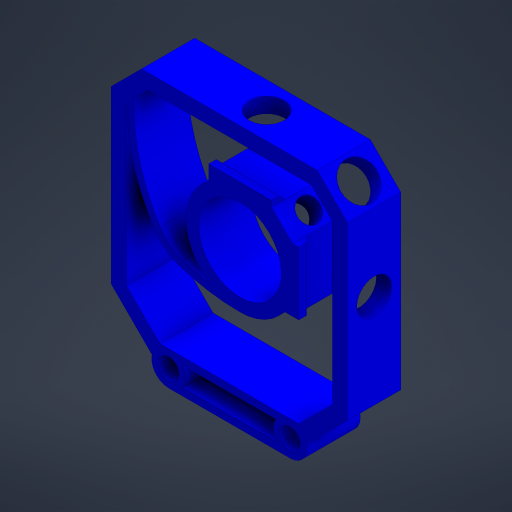
# Autodesk Inventor part: SM05 Lense Holder (V5)
Saved by Autodesk Inventor 2023.4 (Build 274418000, 418)
## iProperties
Created: 2022-07-25
Part Number: SM05 Lense Holder (V5)
Material: Generic
Document SubType Name: Modeling
Designer: xSibe
Density: 1 g/cm^3
Appearance: Plastic Blue
Author: xSibe
Autodesk Inventor part; units mm, degrees
ref_plane "YZ Plane" through (0, 0, 0) normal (1, 0, 0) x (0, 1, 0)
ref_plane "XZ Plane" through (0, 0, 0) normal (0, 1, 0) x (-1, 0, 0)
sketch "Sketch1" plane through (0, 0, 0) normal (0, 0, 1) x (1, 0, 0)
  circle A0 centre (10, 3.85) radius 1.5625
  circle A1 centre (-10, 3.85) radius 1.5625
  line L0 (-16.9, 0) -> (16.9, 0)
  line L1 (16.9, 0) -> (16.9, 7.7)
  line L2 (-16.9, 7.7) -> (16.9, 7.7)
  line L3 (-16.9, 0) -> (-16.9, 7.7)
  circle A2 centre (-10, 3.85) radius 2.8125
  circle A3 centre (10, 3.85) radius 2.8125
  line L4 (-10, 6.6625) -> (10, 6.6625)
  line L5 (10, 1.0375) -> (-10, 1.0375)
  line L6 (-10, 2.2875) -> (10, 2.2875)
  line L7 (-10, 5.4125) -> (10, 5.4125)
  line L8 (-17.05, 7.7) -> (-17.05, 42.1)
  line L9 (17.05, 7.7) -> (17.05, 42.1)
  line L10 (-17.05, 24.9) -> (17.05, 24.9)
  line L11 (0, 24.9) -> (1.767767, 26.667767)
  line L12 (0, 24.9) -> (2.5, 24.9) construction
  circle A4 centre (1.767767, 26.667767) radius 6.78375
  circle A5 centre (1.767767, 26.667767) radius 6.10875
  circle A6 centre (1.767767, 26.667767) radius 8.90875
  line L13 (1.767767, 26.667767) -> (1.767767, 35.576517)
  line L14 (1.767767, 35.576517) -> (1.767767, 35.076517)
  line L15 (-3.419733, 33.826517) -> (6.955267, 33.826517)
  line L16 (6.955267, 33.826517) -> (6.955267, 36.326517)
  line L17 (6.955267, 36.326517) -> (-3.419733, 36.326517)
  line L18 (-3.419733, 36.326517) -> (-3.419733, 33.826517)
  line L19 (-3.419733, 33.826517) -> (6.955267, 36.326517) construction
  line L20 (6.955267, 33.826517) -> (-3.419733, 36.326517) construction
  line L21 (1.767767, 26.667767) -> (8.067204, 32.967204)
  line L22 (8.067204, 32.967204) -> (7.625263, 32.525263)
  line L23 (10.45369, 31.818156) -> (6.918156, 35.35369)
  line L24 (6.918156, 35.35369) -> (4.796836, 33.23237)
  line L25 (4.796836, 33.23237) -> (8.33237, 29.696836)
  line L26 (8.33237, 29.696836) -> (10.45369, 31.818156)
  line L27 (10.45369, 31.818156) -> (4.796836, 33.23237) construction
  line L28 (6.918156, 35.35369) -> (8.33237, 29.696836) construction
  line L29 (10.45369, 31.818156) -> (15.45369, 31.818156) construction
  line L30 (8.926517, 21.480267) -> (8.926517, 31.855267)
  line L31 (8.926517, 31.855267) -> (11.426517, 31.855267)
  line L32 (11.426517, 31.855267) -> (11.426517, 21.480267)
  line L33 (11.426517, 21.480267) -> (8.926517, 21.480267)
  line L34 (1.767767, 35.576517) -> (1.767767, 37.576517)
  line L35 (11.426517, 26.667767) -> (13.426517, 26.667767)
  line L36 (-10.217767, 5.432233) -> (10.217767, 5.432233)
  line L37 (19.467767, 14.682233) -> (19.467767, 39.367767)
  line L38 (14.467767, 44.367767) -> (-14.467767, 44.367767)
  line L39 (-19.467767, 39.367767) -> (-19.467767, 14.682233)
  line L40 (-19.467767, 5.432233) -> (19.467767, 44.367767) construction
  line L41 (19.467767, 5.432233) -> (-19.467767, 44.367767) construction
  line L42 (-10.217767, 5.432233) -> (-19.467767, 14.682233)
  line L43 (10.217767, 5.432233) -> (19.467767, 14.682233)
  line L44 (14.467767, 44.367767) -> (19.467767, 39.367767)
  line L45 (-14.467767, 44.367767) -> (-19.467767, 39.367767)
  line L46 (-15.503301, 46.867767) -> (-21.967767, 40.403301)
  line L47 (-21.967767, 40.403301) -> (-21.967767, 13.646699)
  line L48 (-21.967767, 13.646699) -> (-11.253301, 2.932233)
  line L49 (-11.253301, 2.932233) -> (11.253301, 2.932233)
  line L50 (11.253301, 2.932233) -> (21.967767, 13.646699)
  line L51 (21.967767, 13.646699) -> (21.967767, 40.403301)
  line L52 (21.967767, 40.403301) -> (15.503301, 46.867767)
  line L53 (15.503301, 46.867767) -> (-15.503301, 46.867767)
  line L54 (-13.432233, 41.867767) -> (-16.967767, 38.332233)
  line L55 (-16.967767, 38.332233) -> (-16.967767, 15.717767)
  line L56 (-16.967767, 15.717767) -> (-9.182233, 7.932233)
  line L57 (-9.182233, 7.932233) -> (9.182233, 7.932233)
  line L58 (9.182233, 7.932233) -> (16.967767, 15.717767)
  line L59 (16.967767, 15.717767) -> (16.967767, 38.332233)
  line L60 (16.967767, 38.332233) -> (13.432233, 41.867767)
  line L61 (13.432233, 41.867767) -> (-13.432233, 41.867767)
  line L62 (16.967767, 15.717767) -> (16.967767, 8.646699)
  line L63 (-16.967767, 15.717767) -> (-16.967767, 12.182233)
  line L64 (-19.467767, 14.682233) -> (-19.467767, 11.146699)
  line L65 (19.467767, 14.682233) -> (19.467767, 11.146699)
  circle A7 centre (-10, 3.85) radius 1.705
  circle A8 centre (10, 3.85) radius 1.707
  line L66 (-10, 6.6625) -> (-11.448034, 6.6625)
  line L67 (10, 6.6625) -> (11.448034, 6.6625)
  line L68 (1.767767, 17.759017) -> (-10.732233, 17.759017)
  line L69 (-10.732233, 17.759017) -> (-10.732233, 20.259017)
  arc A9 (-10.732233, 20.259017) -> (1.767767, 17.759017) centre (1.767767, 50.259017) ccw
  arc A10 (-16.967767, 38.332233) -> (-10.732233, 20.259017) centre (12.341914, 38.332233) ccw
  arc A11 (-15.688595, 39.611405) -> (-9.948301, 21.288407) centre (12.341914, 38.332233) ccw
  arc A12 (-9.948301, 21.288407) -> (-3.451418, 19.447938) centre (1.767767, 50.259017) ccw
  line L70 (-10.732233, 20.259017) -> (-12.188467, 22.291105)
  line L71 (-9.948301, 21.288407) -> (-11.376856, 23.340048)
  arc A13 (-12.188467, 22.291105) -> (-8.426288, 19.399152) centre (-6.171148, 26.226005) ccw
  arc A14 (-11.376856, 23.340048) -> (-7.633596, 20.45672) centre (-5.565218, 27.013474) ccw
  point P0 (0, 0)
  point P1 (-7.661464, 2.2875)
  point P2 (-7.661464, 5.4125)
  point P3 (7.661464, 5.4125)
  point P4 (7.661464, 2.2875)
  point P5 (7.341455, 2.932233)
  point P6 (-7.341455, 2.932233)
  point P7 (-11.185824, 6.40029)
  point P8 (11.185824, 6.40029)
  point P9 (-3.419733, 33.910396)
  point P10 (9.010396, 21.480267)
  point P11 (9.010396, 31.855267)
  point P12 (9.581848, 30.946314)
  point P13 (6.046314, 34.481848)
  point P14 (6.955267, 33.910396)
  point P15 (12.751875, 4.430808)
  point P16 (-12.751875, 4.430808)
  point P17 (5.390983, 33.826517)
  point P18 (-2.842005, 34.542767)
  point P19 (9.642767, 22.057995)
  point P20 (8.926517, 30.290983)
  point P21 (10.676517, 26.667767)
  point P22 (10.416579, 31.855267)
  point P23 (9.642767, 31.277539)
  point P24 (6.377539, 34.542767)
  point P25 (1.767767, 35.576517)
  point P26 (6.955267, 35.316579)
  point P27 (8.067204, 32.967204)
  point P28 (-17.05, 12.264466)
  point P29 (16.967767, 24.9)
  point P30 (17.05, 12.264466)
  point P31 (-16.967767, 24.9)
  point P32 (16.967767, 12.182233)
  point P33 (10.499366, 24.9)
  point P34 (-6.963832, 24.9)
  point P35 (-17.05, 41.785534)
  point P36 (17.05, 41.785534)
  point P37 (7.67477, 5.432233)
  point P38 (-7.67477, 5.432233)
  point P39 (12.485534, 7.7)
  point P40 (-12.485534, 7.7)
  point P41 (6.564603, 31.464603)
  dimension "d0" = 1.25
  dimension "d1" = 1.25
  dimension "d2" = 2.5
  dimension "d3" = 45
  dimension "d4" = 13.5675
  dimension "d5" = 0.675
  dimension "d6" = 2.125
  dimension "d7" = 0.5
  dimension "d8" = 10.375
  dimension "d9" = 2.5
  dimension "d10" = 0.625
  dimension "d11" = 5
  dimension "d12" = 135
  dimension "d13" = 3
  dimension "d14" = 2
  dimension "d15" = 2
  dimension "d16" = 38.93553
  dimension "d17" = 38.93553
  dimension "d18" = 9.25
  dimension "d19" = 9.25
  dimension "d20" = 9.25
  dimension "d21" = 9.25
  dimension "d22" = 5
  dimension "d23" = 5
  dimension "d24" = 5
  dimension "d25" = 5
  dimension "d26" = 2.5
  dimension "d46" = 2.5
  dimension "d48" = 0.1425
  dimension "d49" = 0.1445
  dimension "d50" = 12.5
  dimension "d51" = 2.5
  dimension "d52" = 1.25
  dimension "d53" = 2.5
  dimension "d54" = 2.5
  constraints: 132 end point, 28 point on circle, 19 point on line, 14 tangent, 13 centre point, 13 parallel, 10 midpoint, 8 horizontal, 8 perpendicular, 4 symmetric about line, 2 equal length, 2 vertical, 1 coincident, 15 other
  measures "d0" radial gap between concentric circles of A1 A2
  measures "d1" radial gap between concentric circles of A0 A3
  measures "d2" distance of L11.start L11.end
  measures "d3" angle of L12 L11
  measures "d4" diameter of A4
  measures "d5" radial gap between concentric circles of A4 A5
  measures "d6" radial gap between concentric circles of A4 A6
  measures "d7" distance of L13.end L14.end
  measures "d8" distance of L17.end L16.end
  measures "d9" distance of L16.end L15.end
  measures "d10" distance of L21.end L22.end
  measures "d11" distance of L23.start L23.end
  measures "d12" angle of L29 L23
  measures "d13" distance of L24.end L23.end
  measures "d14" distance of L13.end L34.end
  measures "d15" distance of L35.start L35.end
  measures "d16" distance of L40.end L41.end
  measures "d17" distance of L41.end L40.start
  measures "d18" distance of L36.start L40.start
  measures "d19" distance of L39.end L40.start
  measures "d20" distance of L36.end L41.start
  measures "d21" distance of L37.start L41.start
  measures "d22" distance of L38.start L40.end
  measures "d23" distance of L37.end L40.end
  measures "d24" distance of L38.end L41.end
  measures "d25" distance of L39.start L41.end
  measures "d26" distance between parallel lines of L38 L53
  measures "d46" distance between parallel lines of L38 L61
  measures "d48" radial gap between concentric circles of A1 A7
  measures "d49" radial gap between concentric circles of A0 A8
  measures "d50" distance of L68.start L68.end
  measures "d51" distance of L68.end L69.end
  measures "d52" radial gap between concentric circles of A10 A11
  measures "d53" distance of L69.end L70.end
  measures "d54" distance of L71.start L71.end
extrude "Extrusion1" add sketch "Sketch1" along normal mid plane 8.75 contours A8 L49 A3 L7 | L7 A3 L36 A8 | A8 L43 A3 L50 | L50 A3 L6 A8 | A8 L6 A3 L49 | L7 A2 L36 A3 | L36 A3 L43 A8 | A3 L43 L2 L50 | L36 A2 L4 A3 | L7 A7 L36 A2 | A2 L49 A7 L7 | A3 L5 A2 L6 | A3 L67 L43 | L2 L43 L62 L50 | A2 L6 A7 L49 | L36 A7 L42 A2 | A2 L48 A7 L6 | L62 L43 L9 L50 | A2 L42 L66 | L42 A2 L48 L2 | L2 L48 L8 L42 | L62 L59 L10 L9 L43 | L9 L43 L65 L50 | L42 A7 L48 A2 | L42 L8 L10 L55 L63 | L9 L44 L37 L43 | L48 L64 L42 L8 | L42 L39 L45 L8 | L10 L59 L60 L61 L54 L55 L8 L45 L38 L44 L9 | L32 L33 A6 L10 | L10 A6 L26 L23 L31 L32 | A10 L54 A11 L10 | L10 A11 A12 A6 A9 A13 L70 A10 | A6 L33 L30 L10 | L10 L30 L26 A6 | L70 A13 | L30 L33 A6 L10 A4 | L10 A4 L25 L26 L30 | A6 L18 L15 L13 A4 L10 | A14 L71 A11 | L30 L31 A6 L26 | L26 L25 L21 A6 L31 L30 | A6 L31 L23 L26 | L31 A6 L16 L23 | L18 L17 L34 A6 | A6 L13 L15 L18 | L71 A14 A12 | L23 L24 A6 L34 L17 L16 | L16 A6 L24 L23 | L13 L15 L24 L25 A4 | A6 L24 L15 L13 | L25 L24 L15 L16 A6 L21 | L16 L15 L24 A6
sketch "Sketch2" plane through (0, 0, 0) normal (0, 0, 1) x (1, 0, 0)
  circle A0 centre (1.767767, 26.667767) radius 6.78375
  circle A1 centre (1.767767, 26.667767) radius 5.90875
  point P0 (0, 0)
  dimension "d30" = 0.875
  constraints: 1 centre point
  measures "d30" radial gap between concentric circles of A0 A1
extrude "Extrusion2" [suppressed]
sketch "Sketch3" plane through (19.467767, 13.646699, -4.375) normal (1, 0, 0) x (0, 0, -1)
  line L0 (0, 7.833568) -> (-8.75, 7.833568)
  line L1 (0, 18.208568) -> (0, 7.833568)
  line L2 (0, 18.208568) -> (-8.75, 18.208568)
  line L3 (-8.75, 7.833568) -> (-8.75, 18.208568)
  line L4 (-4.375, 18.208568) -> (-4.375, 7.833568)
  circle A0 centre (-4.375, 13.021068) radius 2.875
  point P0 (-4.375, -13.646699)
  dimension "d33" = 5.75
  constraints: 3 midpoint, 2 end point, 1 centre point
  measures "d33" diameter of A0
extrude "Extrusion3" cut sketch "Sketch3" against normal up to surface (2.5 mm away) contours A0 L4 | L4 A0
sketch "Sketch4" plane through (9.848814, 31.855267, -4.375) normal (0, 1, 0) x (1, 0, 0)
  line L0 (1.577703, 0) -> (1.577703, -8.75)
  line L1 (0.567765, 0) -> (1.577703, 0)
  line L2 (1.577703, -8.75) -> (0.567765, -8.75)
  line L3 (1.577703, -8.75) -> (0.567765, -8.75)
  line L4 (0.567765, -8.75) -> (0.567765, -7.5)
  line L5 (0.567765, -7.5) -> (1.577703, -7.5)
  line L6 (1.577703, -7.5) -> (1.577703, -8.75)
  line L7 (1.577703, -7.5) -> (0.567765, -6.490062)
  line L8 (1.577703, -7.5) -> (3.005971, -7.5) construction
  line L9 (0.567765, -4.375) -> (1.577703, -4.375)
  line L10 (1.577703, -1.25) -> (0.567765, -2.259938)
  line L11 (0.567765, 0) -> (0.567765, -8.75)
  point P0 (-9.848814, -4.375)
  point P1 (1.577703, -1.25)
  point P2 (1.577703, -7.5)
  point P3 (0.567765, -6.740062)
  point P4 (0.567765, -2.259938)
  dimension "d36" = 1.25
  dimension "d37" = 135
  constraints: 16 end point, 3 horizontal, 2 midpoint, 2 parallel, 2 symmetric about line, 1 equal length, 1 perpendicular, 1 point on line
  measures "d36" distance of L2.end L4.end
  measures "d37" angle of L8 L7
extrude "Extrusion4" cut sketch "Sketch4" against normal up to surface (10.375 mm away) contours L0 L9 L11 L10 | L0 L7 L11 L9
ref_plane "Work Plane1" through (11.426517, 36.326517, 4.375) normal (0.7071068, -0.7071068, 0) x (0, 0, -1)
mirror "Mirror1" about plane through (11.426517, 36.326517, 4.375) normal (0.7071068, -0.7071068, 0) of "Extrusion3", "Extrusion4"
sketch "Sketch5" plane through (20.2, 38.635534, 4.375) normal (0.7071068, 0.7071068, 0) x (0.7071068, -0.7071068, 0)
  circle A0 centre (-4.571068, 4.375) radius 1.875
  line L0 (-7.018585, 4.375) -> (-2.123551, 4.375)
  circle A1 centre (-4.571068, 4.375) radius 3
  line L1 (-7.018585, 2.259938) -> (-7.018585, 0)
  line L2 (-2.123551, 0) -> (-7.018585, 0)
  line L3 (-2.123551, 8.75) -> (-2.123551, 6.490062)
  line L4 (-7.018585, 8.75) -> (-2.123551, 8.75)
  line L5 (-7.018585, 8.75) -> (-7.018585, 6.490062)
  line L6 (-7.018585, 6.490062) -> (-7.018585, 2.259938)
  line L7 (-2.123551, 2.259938) -> (-2.123551, 0)
  line L8 (-2.123551, 6.490062) -> (-2.123551, 2.259938)
  point P0 (13.035891, 4.375)
  dimension "d40" = 3.75
  dimension "d41" = 6
  constraints: 3 midpoint, 2 centre point, 2 end point, 1 coincident
  measures "d40" diameter of A0
  measures "d41" diameter of A1
extrude "Extrusion5" cut sketch "Sketch5" against normal blind 5 contours L0 A0 | L0 L8 A1 L6 A0 | A0 L0 L6 A1 L8 | A0 L0 | L8 A1 | L6 A1
extrude "Extrusion6" cut sketch "Sketch5" against normal up to next from surface at -11.712296 contours L0 A0 | A0 L0
equation "\"d19\" = d18"
equation "\"d20\" = d18"
equation "\"d21\" = d20"
equation "\"d23\" = d22"
equation "\"d24\" = d22"
equation "\"d25\" = d24"
body "Solid1"
